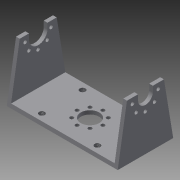
# Autodesk Inventor part: 5
Saved by Autodesk Inventor 2013 (Build 170138000, 138)
## iProperties
Created: 2014-03-05
Part Number: 5
Material: 一般
Document SubType Name: Modeling
Designer: andou
Density: 1 g/cm^3
Author: andou
Title: Bracket
Autodesk Inventor part; units mm, degrees
ref_plane "YZ Plane" through (0, 0, 0) normal (1, 0, 0) x (0, 1, 0)
ref_plane "XZ Plane" through (0, 0, 0) normal (0, 1, 0) x (-1, 0, 0)
ref_plane "XY Plane" through (0, 0, 0) normal (0, 0, 1) x (1, 0, 0)
sketch "スケッチ1" plane through (0, 0, 0) normal (0, 1, 0) x (-1, 0, 0)
  line L0 (30, 14) -> (30, -16)
  line L1 (30, -16) -> (-30, -16)
  line L2 (-30, -16) -> (-30, 14)
  line L3 (28, 14) -> (28, -14)
  line L4 (28, -14) -> (-28, -14)
  line L5 (-28, -14) -> (-28, 14)
  line L6 (-30, 14) -> (-28, 14)
  line L7 (28, 14) -> (30, 14)
  point P0 (0, 0)
  dimension "d0" = 60
  dimension "d2" = 30
  dimension "d3" = 28
  dimension "d4" = 56
  dimension "d5" = 28
  dimension "d6" = 14
  dimension "d7" = 30
  dimension "d8" = 16
  dimension "d9" = 28
  dimension "d11" = 28
  constraints: 16 end point, 4 parallel, 2 horizontal, 2 perpendicular
  measures "d0" distance of L0.end L1.end
  measures "d2" distance of L1.end L2.end
  measures "d3" distance of L4.end L5.end
  measures "d4" distance of L3.end L4.end
  measures "d5" distance from line of point (0, 0) L5
  measures "d6" distance from line of point (0, 0) L4
  measures "d7" distance from line of point (0, 0) L0
  measures "d8" distance from line of point (0, 0) L1
  measures "d9" distance of L3.start L3.end
  measures "d11" distance from line of L3 point (0, 0)
extrude "押し出し1" add sketch "スケッチ1" along normal blind 30
sketch "スケッチ2" plane through (30, 0, 14) normal (1, 0, 0) x (0, 0, -1)
  line L0 (30, 0) -> (30, 30) projected
  line L1 (0, 0) -> (0, 30) projected
  line L2 (30, 30) -> (0, 25)
  line L3 (30, 0) -> (0, 5)
  point P0 (14, 0)
  dimension "d75" = 20
  constraints: 4 end point, 2 point on line, 1 equal length
  measures "d75" distance of L2.end L3.end
extrude "押し出し2" cut sketch "スケッチ2" against normal blind 60 keep common part
sketch "スケッチ3" plane through (30, 0, -16) normal (1, 0, 0) x (0, 0, -1)
  line L0 (-30, 5) -> (-30, 25) projected
  line L1 (0, 0) -> (0, 30) projected
  arc A0 (-27, 11) -> (-27, 19) centre (-27, 15) ccw
  line L2 (-27, 19) -> (-30, 19)
  line L3 (-27, 11) -> (-30, 11)
  point P0 (-16, 0)
  dimension "d20" = 8
  dimension "d79" = 3
  dimension "d82" = 15
  constraints: 4 end point, 2 perpendicular, 2 point on circle, 2 point on line, 2 tangent, 1 centre point
  measures "d20" diameter of A0
  measures "d79" distance from line of L0 A0.centre
  measures "d82" vertical distance of A0.centre L1.start
extrude "押し出し3" cut sketch "スケッチ3" against normal blind 2
sketch "スケッチ4" plane through (-30, 0, -16) normal (-1, 0, 0) x (0, 0, 1)
  line L0 (30, 5) -> (30, 25) projected
  arc A0 (27, 20) -> (27, 10) centre (27, 15) ccw
  line L1 (27, 20) -> (30, 20)
  line L2 (27, 10) -> (30, 10)
  point P0 (16, 0)
  point P1 (0, 30)
  dimension "d25" = 10
  dimension "d80" = 3
  dimension "d81" = 15
  constraints: 4 end point, 2 perpendicular, 2 point on circle, 2 point on line, 2 tangent, 1 centre point
  measures "d25" diameter of A0
  measures "d80" distance from line of L0 A0.centre
  measures "d81" vertical distance of point (0, 30) A0.centre
extrude "押し出し4" cut sketch "スケッチ4" against normal blind 2
sketch "スケッチ7" plane through (30, 0, -16) normal (0, 0, -1) x (-1, 0, 0)
  line L0 (0, 0) -> (60, 0) projected
  line L1 (0, 0) -> (0, 30) projected
  circle A0 centre (30, 15) radius 5
  point P0 (30, 0)
  dimension "d45" = 10
  dimension "d47" = 15
  dimension "d48" = 30
  constraints: 1 centre point
  measures "d45" diameter of A0
  measures "d47" distance from line of A0.centre L0
  measures "d48" distance from line of L1 A0.centre
hole "穴2" at (0, 15, -16) direction (0, 0, 1) diameter 10 end through all
sketch "スケッチ8" plane through (30, 0, -16) normal (0, 0, -1) x (-1, 0, 0)
  circle A0 centre (30, 15) radius 5 projected
  line L0 (0, 0) -> (0, 30) projected
  circle A1 centre (30, 22) radius 1
  line L1 (30, 15) -> (30, 22)
  point P0 (30, 0)
  dimension "d56" = 2
  dimension "d58" = 0
  dimension "d62" = 7
  constraints: 2 end point, 1 centre point
  measures "d56" diameter of A1
  measures "d58" angle of L0 L1
  measures "d62" distance of L1.end L1.start
hole "穴3" at (0, 22, -16) direction (0, 0, 1) diameter 2 end through all
pattern_circular "円形状パターン2" count 8 over 360 about axis through (0, 15, 57.4847) along (0, 0, -1) of "穴2", "穴3"
sketch "スケッチ9" plane through (30, 0, -16) normal (1, 0, 0) x (0, 0, -1)
  arc A0 (-27, 11) -> (-27, 19) centre (-27, 15) ccw projected
  line L0 (-30, 19) -> (-30, 25) projected
  circle A1 centre (-27, 22) radius 1
  line L1 (-27, 15) -> (-27, 22)
  point P0 (-16, 0)
  dimension "d83" = 2
  dimension "d85" = 7
  constraints: 2 end point, 1 centre point, 1 parallel
  measures "d83" diameter of A1
  measures "d85" distance of L1.start L1.end
hole "穴4" at (30, 22, 11) direction (-1, 0, 0) diameter 2 end through all
pattern_circular "円形状パターン3" count 5 over 180 about axis through (30, 15, 11) along (-1, 0, 0) of "穴4"
sketch "スケッチ10" plane through (30, 0, -16) normal (0, 0, -1) x (-1, 0, 0)
  circle A0 centre (30, 15) radius 5 projected
  line L0 (0, 30) -> (60, 30) projected
  circle A1 centre (15, 26) radius 1.5
  circle A2 centre (15, 4) radius 1.5
  circle A3 centre (45, 4) radius 1.5
  circle A4 centre (45, 26) radius 1.5
  point P0 (30, 0)
  dimension "d96" = 30
  dimension "d98" = 22
  dimension "d99" = 4
  dimension "d100" = 22
  dimension "d101" = 4
  dimension "d102" = 30
  dimension "d103" = 15
  dimension "d104" = 15
  dimension "d105" = 3
  constraints: 4 centre point, 3 equal radius
  measures "d96" distance of A4.centre A1.centre
  measures "d98" distance of A1.centre A2.centre
  measures "d99" distance from line of L0 A1.centre
  measures "d100" distance of A4.centre A3.centre
  measures "d101" distance from line of L0 A4.centre
  measures "d102" distance of A3.centre A2.centre
  measures "d103" horizontal distance of A0.centre A2.centre
  measures "d104" horizontal distance of A0.centre A1.centre
  measures "d105" diameter of A4
hole "穴5" at (15, 4, -16) at (-15, 4, -16) at (-15, 26, -16) at (15, 26, -16) direction (0, 0, 1) diameter 3 end through all
thread "ねじ5" size "M3x0.5" class "6H" standard "ANSI Metric M Profile" full length
thread "ねじ6" size "M3x0.5" class "6H" standard "ANSI Metric M Profile" full length
thread "ねじ7" size "M3x0.5" class "6H" standard "ANSI Metric M Profile" full length
thread "ねじ8" size "M3x0.5" class "6H" standard "ANSI Metric M Profile" full length
